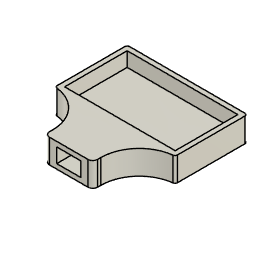
zrcatko male (Autodesk Fusion 360 design; units mm, degrees)
Autodesk Fusion 360 part; units mm, degrees
sketch "Sketch1" plane through (0, 0, 0) normal (0, 0, 1) x (1, 0, 0)
  line L0 (-12.5, -7.5) -> (12.5, -7.5)
  line L1 (12.5, -7.5) -> (12.5, 7.5)
  line L2 (12.5, 7.5) -> (-12.5, 7.5)
  line L3 (-12.5, 7.5) -> (-12.5, -7.5)
  line L4 (-11.5, 6.5) -> (11.5, 6.5)
  line L5 (11.5, 6.5) -> (11.5, -6.5)
  line L6 (11.5, -6.5) -> (-11.5, -6.5)
  line L7 (-11.5, -6.5) -> (-11.5, 6.5)
  line L8 (-5, -7.5) -> (5, -7.5)
  line L9 (5, -7.5) -> (5, -17.15)
  line L10 (5, -17.15) -> (-5, -17.15)
  line L11 (-5, -17.15) -> (-5, -7.5)
  dimension "d1" = 15
  dimension "d2" = 7.5
  dimension "d3" = 25
  dimension "d4" = 12.5
  dimension "d5" = 23
  dimension "d6" = 13
  dimension "d7" = 1
  dimension "d8" = 1
  dimension "d10" = 10
  dimension "d11" = 5
  dimension "d30" = 9.65
  constraint horizontal L0
  constraint vertical L1
  constraint horizontal L2
  constraint vertical L3
  constraint horizontal L4
  constraint vertical L5
  constraint horizontal L6
  constraint vertical L7
  constraint horizontal L8
  constraint vertical L9
  constraint horizontal L10
  constraint vertical L11
  constraint coincident L0 L8.start
  measures "d1" distance of L0.start L2.end
  measures "d2" distance of origin L0
  measures "d3" distance of L1.end L2.end
  measures "d4" distance of origin L1
  measures "d5" distance of L4.start L4.end
  measures "d6" distance of L4.start L6.end
  measures "d7" distance of L2 L4
  measures "d8" distance of L1 L5
  measures "d10" distance of L9.end L10.end
  measures "d11" distance of origin L11
  measures "d30" distance of L8 L10
extrude "Extrude1" add sketch "Sketch1" along normal blind 5
fillet "Fillet1" radius 8 2 edges at (-5, -7.5, 2.5) (5, -7.5, 2.5)
fillet "Fillet2" radius 0.5 4 edges at (-12.5, -7.5, 2.5) (-12.5, 7.5, 2.5) (12.5, 7.5, 2.5) (12.5, -7.5, 2.5)
sketch "Sketch2" plane through (0, -17.15, 0) normal (0, -1, 0) x (1, 0, 0)
  line L0 (-5, 0) -> (5, 0)
  line L1 (5, 0) -> (5, 5)
  line L2 (5, 5) -> (-5, 5)
  line L3 (-5, 5) -> (-5, 0)
  line L4 (-2.5, 4) -> (2.5, 4)
  line L5 (2.5, 4) -> (2.5, 1)
  line L6 (2.5, 1) -> (-2.5, 1)
  line L7 (-2.5, 1) -> (-2.5, 4)
  dimension "d20" = 5
  dimension "d21" = 2.5
  dimension "d22" = 1
  dimension "d23" = 3
  constraint horizontal L4
  constraint vertical L5
  constraint horizontal L6
  constraint vertical L7
  measures "d20" distance of L4.start L4.end
  measures "d21" distance of L3 L7
  measures "d22" distance of L2 L4
  measures "d23" distance of L4.end L5.end
extrude "Extrude2" cut sketch "Sketch2" against normal blind 5 contours L4 L5 L6 L7
fillet "Fillet3" radius 1 2 edges at (-5, -17.15, 2.5) (5, -17.15, 2.5)
extrude "Extrude3" add sketch "Sketch1" along normal blind 2 contours L4 L5 L6 L7
